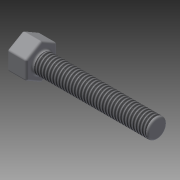
# Autodesk Inventor part: SzenzorCsavar5os
Saved by Autodesk Inventor 2015 SP1 (Build 190203100, 203)
## iProperties
Created: 2014-09-14
Part Number: SzenzorCsavar5os
Material: Generic
Document SubType Name: Modeling
Designer: laca
Density: 1 g/cm^3
Appearance: Default
Mass: 0.862985 g
Surface Area: 7.00139 cm^2
Volume: 0.862985 cm^3
Author: laca
Autodesk Inventor part; units mm, degrees
ref_plane "YZ Plane" through (0, 0, 0) normal (1, 0, 0) x (0, 1, 0)
ref_plane "XZ Plane" through (0, 0, 0) normal (0, 1, 0) x (-1, 0, 0)
ref_plane "XY Plane" through (0, 0, 0) normal (0, 0, 1) x (1, 0, 0)
sketch "Sketch1" plane through (0, 0, 0) normal (1, 0, 0) x (0, 1, 0)
  circle A0 centre (0, 0) radius 2.5
  line L0 (2.3039, 4.0032) -> (4.6188, 0.0063)
  line L1 (4.6188, 0.0063) -> (2.3149, -3.9968)
  line L2 (2.3149, -3.9968) -> (-2.3039, -4.0032)
  line L3 (-2.3039, -4.0032) -> (-4.6188, -0.0063)
  line L4 (-4.6188, -0.0063) -> (-2.3149, 3.9968)
  line L5 (-2.3149, 3.9968) -> (2.3039, 4.0032)
  dimension "d0" = 5
  dimension "d1" = 8
  constraints: 12 end point, 2 coincident, 1 centre point, 13 other
  measures "d0" diameter of A0
  measures "d1" distance between parallel lines of L3 L0
extrude "Extrusion1" add sketch "Sketch1" along normal blind 30 contours A0
extrude "Extrusion2" add sketch "Sketch1" against normal blind 5 contours A0 | L0 L1 L2 L3 L4 L5
thread "Thread1" size "M5x0.8" class "6g" standard "ANSI Metric M Profile" full length
fillet "Fillet1" radius 0.5 6 edges at (-2.5, 2.3039, 4.0032) (-2.5, 4.6188, 0.0063) (-2.5, -2.3149, 3.9968) (-2.5, -4.6188, -0.0063) (-2.5, -2.3039, -4.0032) (-2.5, 2.3149, -3.9968)
fillet "Fillet2" radius 0.5 24 edges at (-5, -4.5414, -0.0062) (-5, -3.4668, 1.9953) (-5, -2.2761, 3.9299) (-5, -0.0055, 4) (-5, 2.2653, 3.9361) (-5, 3.4614, 2.0047) (-5, 4.5414, 0.0062) (-5, 3.4668, -1.9953) (-5, 2.2761, -3.9299) (-5, 0.0055, -4) (-5, -2.2653, -3.9361) (-5, -3.4614, -2.0047) (0, -4.5414, -0.0062) (0, -3.4668, 1.9953) (0, -2.2761, 3.9299) (0, -0.0055, 4) (0, 2.2653, 3.9361) (0, 3.4614, 2.0047) (0, 4.5414, 0.0062) (0, 3.4668, -1.9953) (0, 2.2761, -3.9299) (0, 0.0055, -4) (0, -2.2653, -3.9361) (0, -3.4614, -2.0047)
fillet "Fillet3" radius 0.5 2 edges at (0, -2.5, 0) (30, -2.5, 0)
body "Solid1"
